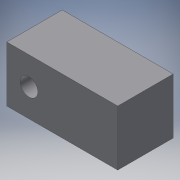
# Autodesk Inventor part: bracket3
Saved by Autodesk Inventor 2018.2 (Build 222227000, 227)
## iProperties
Created: 2018-03-19
Part Number: bracket3
Material: 一般
Document SubType Name: Modeling
Designer: ku_sk
Density: 1 g/cm^3
Appearance: 既定
Author: ku_sk
Autodesk Inventor part; units mm, degrees
ref_plane "YZ Plane" through (0, 0, 0) normal (1, 0, 0) x (0, 1, 0)
ref_plane "XZ Plane" through (0, 0, 0) normal (0, 1, 0) x (-1, 0, 0)
ref_plane "XY Plane" through (0, 0, 0) normal (0, 0, 1) x (1, 0, 0)
sketch "スケッチ1" plane through (0, 0, 0) normal (1, 0, 0) x (0, 1, 0)
  line L0 (-12.5, 12.5) -> (12.5, 12.5)
  line L1 (12.5, 12.5) -> (12.5, -12.5)
  line L2 (12.5, -12.5) -> (-12.5, -12.5)
  line L3 (-12.5, -12.5) -> (-12.5, 12.5)
  line L4 (-12.5, 12.5) -> (12.5, -12.5) construction
  line L5 (12.5, 12.5) -> (-12.5, -12.5) construction
  point P0 (0, 0)
  dimension "d0" = 25
  dimension "d1" = 25
  constraints: 12 end point, 2 midpoint, 2 parallel, 1 horizontal, 1 perpendicular
  measures "d0" distance of L0.start L0.end
  measures "d1" distance of L0.end L1.end
extrude "押し出し1" add sketch "スケッチ1" along normal blind 50
sketch "スケッチ2" plane through (0, 12.5, 12.5) normal (0, 1, 0) x (1, 0, 0)
  circle A0 centre (10, 12.5) radius 6
  line L0 (0, 0) -> (0, 25) projected
  line L1 (0, 0) -> (50, 0) projected
  point P0 (0, 12.5)
  dimension "d4" = 12
  dimension "d5" = 10
  dimension "d6" = 12.5
  constraints: 1 centre point
  measures "d4" diameter of A0
  measures "d5" distance from line of L0 A0.centre
  measures "d6" distance from line of A0.centre L1
extrude "押し出し2" cut sketch "スケッチ2" against normal through all
equation "\"d1\" = d0"
